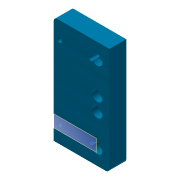
# Autodesk Inventor part: RightAngleMotorMountExtensionArm
Saved by Autodesk Inventor 2018 (Build 220112000, 112)
## iProperties
Created: 2019-01-17
Part Number: RightAngleMotorMountExtensionArm
Material: Generic
Document SubType Name: Modeling
Designer: ball
Density: 1 g/cm^3
Appearance: Default
Author: ball
Autodesk Inventor part; units mm, degrees
ref_plane "YZ Plane" through (0, 0, 0) normal (1, 0, 0) x (0, 1, 0)
ref_plane "XZ Plane" through (0, 0, 0) normal (0, 1, 0) x (-1, 0, 0)
ref_plane "XY Plane" through (0, 0, 0) normal (0, 0, 1) x (1, 0, 0)
ref_plane "Work Plane1" through (-2.3114, 87.1581, 14.5288) normal (0, 0, -1) x (-1, 0, 0)
sketch "Sketch1" plane through (-2.3114, 87.1581, 14.5288) normal (0, 0, -1) x (-1, 0, 0)
  line L0 (0, -9.525) -> (33.4772, -9.525) construction
  line L1 (35.1536, 0) -> (35.1536, -9.525) construction
  line L2 (0, 62.419) -> (33.4772, 62.419) construction
  line L3 (-12.7, -19.685) -> (-12.7, 72.579)
  arc A0 (30.0098, 55.9153) -> (28.8277, 56.5778) centre (30.209, 57.6565) ccw construction
  arc A1 (30.0098, -6.5037) -> (28.8277, -5.8412) centre (30.209, -4.7625) ccw construction
  spline S0 degree 3 poles (-36.5707, 76.7108) (-36.5399, 76.774) (-36.5004, 76.8533) (-36.4067, 77.0384) (-36.3532, 77.143) (-36.2191, 77.4029) (-36.1252, 77.5838) (-35.9667, 77.8845) (-35.9172, 77.9778) (-35.7665, 78.2605) (-35.6659, 78.447) (-35.4766, 78.7937) (-35.4006, 78.9307) (-35.2724, 79.1587) (-35.2158, 79.2566) (-35.126, 79.4049) (-35.0957, 79.4501) (-35.0767, 79.4671) (-35.0747, 79.4643) (-35.0811, 79.4361) (-35.0968, 79.3935) (-35.1824, 79.2047) (-35.234, 79.0957) (-35.3802, 78.7956) (-35.4651, 78.6264) (-35.5969, 78.3654) (-35.6729, 78.2163) (-35.8204, 77.9297) (-35.8907, 77.794) (-36.0446, 77.5001) (-36.107, 77.3829) (-36.1471, 77.3082) knots 0.000001 0.000001 0.000001 0.000001 0.04651 0.04651 0.092381 0.092381 0.150569 0.150569 0.176245 0.176245 0.228297 0.228297 0.280311 0.280311 0.337729 0.337729 0.399083 0.399083 0.42945 0.42945 0.476927 0.476927 0.513851 0.513851 0.562369 0.562369 0.621068 0.621068 0.675896 0.675896 0.74783 0.74783 0.74783 0.74783 construction
  spline S1 degree 3 poles (-36.5707, 14.2918) (-36.5399, 14.355) (-36.5004, 14.4343) (-36.4067, 14.6194) (-36.3532, 14.724) (-36.2191, 14.9839) (-36.1252, 15.1648) (-35.9667, 15.4655) (-35.9172, 15.5588) (-35.7665, 15.8415) (-35.6659, 16.028) (-35.4766, 16.3747) (-35.4006, 16.5117) (-35.2724, 16.7397) (-35.2158, 16.8376) (-35.126, 16.9859) (-35.0957, 17.0311) (-35.0767, 17.0481) (-35.0747, 17.0453) (-35.0811, 17.0171) (-35.0968, 16.9745) (-35.1824, 16.7857) (-35.234, 16.6767) (-35.3802, 16.3766) (-35.4651, 16.2074) (-35.5969, 15.9464) (-35.6729, 15.7973) (-35.8204, 15.5107) (-35.8907, 15.375) (-36.0446, 15.0811) (-36.107, 14.9639) (-36.1471, 14.8892) knots 0.000001 0.000001 0.000001 0.000001 0.04651 0.04651 0.092381 0.092381 0.150569 0.150569 0.176245 0.176245 0.228297 0.228297 0.280311 0.280311 0.337729 0.337729 0.399083 0.399083 0.42945 0.42945 0.476927 0.476927 0.513851 0.513851 0.562369 0.562369 0.621068 0.621068 0.675896 0.675896 0.74783 0.74783 0.74783 0.74783 construction
  circle A2 centre (30.209, -4.7625) radius 1.9685
  circle A3 centre (30.209, 57.6565) radius 1.9685
  arc A4 (3.0691, -6.5037) -> (1.8869, -5.8412) centre (3.2682, -4.7625) ccw construction
  arc A5 (3.0691, 55.9153) -> (1.8869, 56.5778) centre (3.2682, 57.6565) ccw construction
  circle A6 centre (3.2682, 57.6565) radius 1.9685
  circle A7 centre (3.2682, -4.7625) radius 1.9685
  line L4 (35.1536, -19.685) -> (-12.7, -19.685)
  line L5 (35.1536, 72.579) -> (-12.7, 72.579)
  line L6 (35.1536, -19.685) -> (35.1536, 72.579)
  point P0 (-2.3114, -87.1581)
  point P1 (-12.7, 62.419)
  dimension "d0" = 3.937
  dimension "d1" = 3.937
  dimension "d4" = 3.937
  dimension "d5" = 3.937
  constraints: 14 end point, 8 centre point, 8 point on circle, 4 coincident, 2 horizontal, 2 point on line, 2 vertical, 30 other
  measures "d0" diameter of A2
  measures "d1" diameter of A3
  measures "d4" diameter of A6
  measures "d5" diameter of A7
ref_plane "Work Plane2" through (-72.402, 8.8416, 0) normal (0, 0, 1) x (1, 0, 0)
ref_plane "Work Plane3" through (-84.9315, 9.3639, 0) normal (0, 0, 1) x (1, 0, 0)
extrude "Extrusion2" add sketch "Sketch1" along normal up to surface (14.5288 mm away)
sketch "Sketch2" plane through (10.3886, 77.6331, 0) normal (0, 0, -1) x (-1, 0, 0)
  circle A0 centre (42.909, 4.7625) radius 1.9685 projected
  circle A1 centre (42.909, 4.7625) radius 1.9685
  circle A2 centre (42.909, 67.1815) radius 1.9685 projected
  circle A3 centre (42.909, 67.1815) radius 1.9685
  circle A4 centre (15.9682, 4.7625) radius 1.9685 projected
  circle A5 centre (15.9682, 4.7625) radius 1.9685
  circle A6 centre (15.9682, 67.1815) radius 1.9685 projected
  circle A7 centre (15.9682, 67.1815) radius 1.9685
  point P0 (10.3886, -77.6331)
  dimension "d12" = 3.937
  dimension "d13" = 3.937
  dimension "d14" = 3.937
  dimension "d15" = 3.937
  constraints: 4 centre point, 4 coincident
  measures "d12" diameter of A1
  measures "d13" diameter of A3
  measures "d14" diameter of A5
  measures "d15" diameter of A7
hole "Hole1" at (-5.5796, 144.8146, 0) at (-32.5204, 144.8146, 0) at (-32.5204, 82.3956, 0) at (-5.5796, 82.3956, 0) direction (0, 0, 1) diameter 3.937 end through all counterbore diameter 8.89 counterbore depth 5.08
sketch "Sketch3" plane through (-2.3114, 87.1581, 14.5288) normal (0, 0, 1) x (1, 0, 0)
  arc A0 (3.5282, -17.9067) -> (2.2941, -18.3979) centre (2.3114, -16.6454) ccw construction
  arc A1 (3.5282, 9.034) -> (2.2941, 8.5429) centre (2.3114, 10.2954) ccw construction
  arc A2 (3.5282, 41.3373) -> (2.2941, 40.8461) centre (2.3114, 42.5986) ccw construction
  arc A3 (3.5282, 68.278) -> (2.2941, 67.7869) centre (2.3114, 69.5394) ccw construction
  circle A4 centre (2.3114, -16.6454) radius 1.9685
  circle A5 centre (2.3114, 10.2954) radius 1.9685
  circle A6 centre (2.3114, 42.5986) radius 1.9685
  circle A7 centre (2.3114, 69.5394) radius 1.9685
  point P0 (2.3114, -87.1581)
  dimension "d37" = 3.937
  dimension "d38" = 3.937
  dimension "d39" = 3.937
  dimension "d40" = 3.937
  constraints: 8 centre point, 8 point on circle, 4 coincident, 16 other
  measures "d37" diameter of A4
  measures "d38" diameter of A5
  measures "d39" diameter of A6
  measures "d40" diameter of A7
hole "Hole2" at (0, 70.5127, 14.5288) at (0, 97.4535, 14.5288) at (0, 129.7567, 14.5288) at (0, 156.6975, 14.5288) direction (0, 0, -1) diameter 3.937 end through all counterbore diameter 8.89 counterbore depth 5.334
fillet "Fillet1" radius 3.175 2 edges at (10.3886, 67.4731, 7.2644) (-37.465, 159.7371, 7.2644)
body "Solid2"
